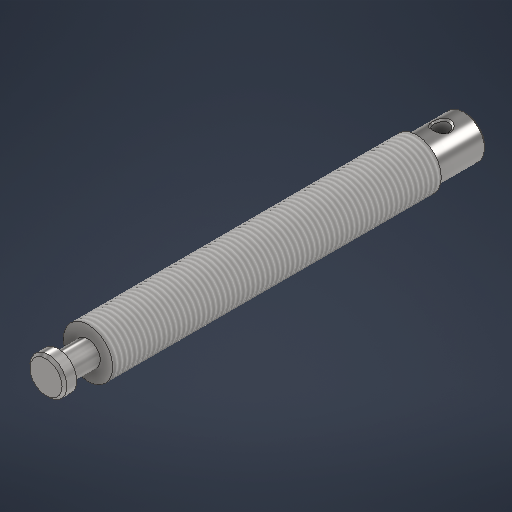
# Autodesk Inventor part: Part8
Saved by Autodesk Inventor 2026.2 (Build 302298010, 298A)
## iProperties
Created: 2026-03-22
Part Number: Part8
Material: Generic
Document SubType Name: Modeling
Designer: Mlinč
Density: 1 g/cm^3
Appearance: Default
Author: Mlinč
Autodesk Inventor part; units mm, degrees
ref_plane "YZ Plane" through (0, 0, 0) normal (1, 0, 0) x (0, 1, 0)
ref_plane "XZ Plane" through (0, 0, 0) normal (0, 1, 0) x (-1, 0, 0)
ref_plane "XY Plane" through (0, 0, 0) normal (0, 0, 1) x (1, 0, 0)
sketch "Sketch1" plane through (0, 0, 0) normal (1, 0, 0) x (0, 1, 0)
  line L0 (0, 0) -> (0, -170)
  line L1 (0, 0) -> (6.5, 0)
  line L2 (6.5, 0) -> (7.5, -1)
  line L3 (7.5, -1) -> (7.5, -5)
  line L4 (7.5, -5) -> (5, -5)
  line L5 (5, -5) -> (5, -17)
  line L6 (5, -17) -> (10, -17)
  line L7 (10, -17) -> (10, -150)
  line L8 (10, -150) -> (8.5, -150)
  line L9 (8.5, -150) -> (8.5, -169)
  line L10 (7.5, -170) -> (0, -170)
  line L11 (8.5, -169) -> (7.5, -170)
  point P0 (8.5, -170)
  dimension "d0" = 170
  dimension "d1" = 17
  dimension "d2" = 20
  dimension "d3" = 10
  dimension "d4" = 15
  dimension "d5" = 5
  dimension "d6" = 1
  dimension "d7" = 1
  dimension "d8" = 12
  dimension "d9" = 20
  dimension "d10" = 1
  dimension "d11" = 1
  constraints: 24 end point, 8 perpendicular, 2 point on line, 1 coincident, 1 horizontal, 1 vertical
  measures "d0" distance of L0.start L0.end
  measures "d1" diameter of L9 L0
  measures "d2" diameter of L7 L0
  measures "d3" diameter of L5 L0
  measures "d4" diameter of L3 L0
  measures "d5" distance between parallel lines of L1 L4
  measures "d6" distance from line of L1 L2.end
  measures "d7" distance from line of L3 L1.end
  measures "d8" distance between parallel lines of L6 L4
  measures "d9" distance between parallel lines of L10 L8
  measures "d10" distance of L9.end point (8.5, -170)
  measures "d11" distance of L10.start point (8.5, -170)
revolve "Revolution1" add sketch "Sketch1" angle 360 about axis through (0, 0, 0) along (0, 0, -1)
sketch "Sketch2" plane through (0, 0, 0) normal (0, 1, 0) x (-1, 0, 0)
  circle A0 centre (0, -160) radius 3
  line L0 (-7.5, -170) -> (7.5, -170) projected
  point P0 (0, 0)
  dimension "d13" = 6
  dimension "d14" = 10
  constraints: 1 centre point, 1 vertical alignment
  measures "d13" diameter of A0
  measures "d14" distance from line of L0 A0.centre
extrude "Extrusion1" cut sketch "Sketch2" along normal through all both and the other way through all
chamfer "Chamfer1" distance 0.75 angle 45 4 edges at (3, 7.953, -159.9995) (-2.2741, 8.1902, -158.0433) (-2.2734, 8.1903, -161.9575) (3, -7.953, -160.0011)
thread "Thread1" size "TR20x2" class "7e" standard "ISO Metric Trapezoidal Threads" full length
equation "\"d11\" = d10"
body "Solid1"
